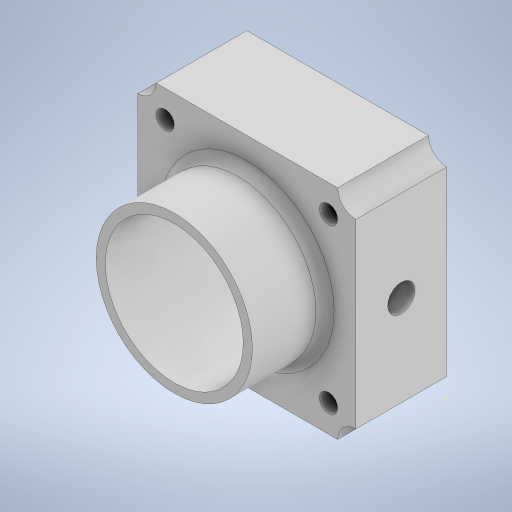
# Autodesk Inventor part: Base
Saved by Autodesk Inventor 2023 (Build 270158000, 158)
## iProperties
Created: 2023-07-24
Part Number: Base
Material: Generic
Document SubType Name: Modeling
Designer: User
Density: 1 g/cm^3
Appearance: Default
Author: User
Autodesk Inventor part; units mm, degrees
ref_plane "YZ Plane" through (0, 0, 0) normal (1, 0, 0) x (0, 1, 0)
ref_plane "XZ Plane" through (0, 0, 0) normal (0, 1, 0) x (-1, 0, 0)
ref_plane "XY Plane" through (0, 0, 0) normal (0, 0, 1) x (1, 0, 0)
sketch "Sketch4" plane through (0, 0, 0) normal (0, 0, 1) x (1, 0, 0)
  line L0 (0, 0) -> (120, 0)
  line L1 (120, 0) -> (120, 120)
  line L2 (120, 120) -> (0, 120)
  line L3 (0, 120) -> (0, 0)
  dimension "d11" = 120
  dimension "d12" = 120
  constraints: 8 end point, 2 parallel, 1 horizontal, 1 perpendicular
  measures "d11" distance of L0.start L0.end
  measures "d12" distance of L2.end L0.start
extrude "Extrusion1" add sketch "Sketch4" along normal blind 50
sketch "Sketch5" plane through (0, 0, 50) normal (0, 0, 1) x (1, 0, 0)
  point P0 (0, 0)
sketch "Sketch6" plane through (0, 0, 50) normal (0, 0, 1) x (1, 0, 0)
  circle A0 centre (60, 60) radius 43
  line L0 (120, 0) -> (120, 120) projected
  line L1 (120, 120) -> (0, 120) projected
  point P0 (0, 0)
  dimension "d15" = 86
  dimension "d16" = 60
  dimension "d17" = 60
  constraints: 1 centre point
  measures "d15" diameter of A0
  measures "d16" distance from line of L0 A0.centre
  measures "d17" distance from line of L1 A0.centre
extrude "Extrusion2" add sketch "Sketch6" along normal blind 40 and the other way blind 20
fillet "Fillet1" radius 5 1 edges at (17, 60, 50)
sketch "Sketch7" plane through (60, 60, 90) normal (0, 0, 1) x (1, 0, 0)
  circle A0 centre (0, 0) radius 43 projected
  point P0 (-60, -60)
  constraints: 1 coincident
hole "Hole1" at (60, 60, 90) direction (0, 0, -1) diameter 76 end through all
sketch "Sketch8" plane through (120, 0, 0) normal (1, 0, 0) x (0, 0, -1)
  point P0 (0, 0)
sketch "Sketch9" plane through (120, 0, 0) normal (1, 0, 0) x (0, 0, -1)
  line L0 (0, 120) -> (0, 0) projected
  line L1 (0, 120) -> (-50, 120) projected
  point P0 (-25, 60)
  dimension "d30" = 25
  dimension "d38" = 60
  measures "d30" distance from line of L0 point (-25, 60)
  measures "d38" distance from line of L1 point (-25, 60)
hole "Hole2" at (120, 60, 25) direction (-1, 0, 0) diameter 15 end through all
fillet "Fillet2" radius 10 4 edges at (120, 120, 25) (0, 120, 25) (120, 0, 25) (0, 0, 25) inverted yes
sketch "Sketch10" plane through (0, 0, 50) normal (0, 0, 1) x (1, 0, 0)
  line L0 (120, 10) -> (120, 110) projected
  line L1 (110, 120) -> (10, 120) projected
  line L2 (10, 0) -> (110, 0) projected
  line L3 (0, 110) -> (0, 10) projected
  point P0 (0, 0)
  point P1 (105, 105)
  point P2 (105, 15)
  point P3 (15, 15)
  point P4 (15, 105)
  dimension "d40" = 15
  dimension "d48" = 15
  dimension "d49" = 15
  dimension "d50" = 15
  dimension "d51" = 15
  dimension "d52" = 15
  dimension "d53" = 15
  dimension "d54" = 15
  measures "d40" distance from line of L0 point (105, 105)
  measures "d48" distance from line of L1 point (105, 105)
  measures "d49" distance from line of L0 point (105, 15)
  measures "d50" distance from line of L2 point (105, 15)
  measures "d51" distance from line of L2 point (15, 15)
  measures "d52" distance from line of L3 point (15, 15)
  measures "d53" distance from line of L1 point (15, 105)
  measures "d54" distance from line of L3 point (15, 105)
hole "Hole3" at (105, 105, 50) at (105, 15, 50) at (15, 15, 50) at (15, 105, 50) direction (0, 0, -1) diameter 10 end through all
body "Solid1"
